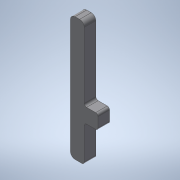
# Autodesk Inventor part: Zlifter
Saved by Autodesk Inventor 2020 (Build 240168000, 168)
## iProperties
Created: 2019-05-25
Part Number: Zlifter
Material: Generic
Document SubType Name: Modeling
Designer: LillaHunden
Density: 1 g/cm^3
Appearance: Default
Author: LillaHunden
Autodesk Inventor part; units mm, degrees
ref_plane "YZ Plane" through (0, 0, 0) normal (1, 0, 0) x (0, 1, 0)
ref_plane "XZ Plane" through (0, 0, 0) normal (0, 1, 0) x (-1, 0, 0)
ref_plane "XY Plane" through (0, 0, 0) normal (0, 0, 1) x (1, 0, 0)
sketch "Sketch1" plane through (0, 0, 0) normal (0, 0, 1) x (1, 0, 0)
  circle A0 centre (-14.5473, 15.1065) radius 1.65 construction
  circle A1 centre (16.4527, 46.1065) radius 1.65 construction
  circle A2 centre (-14.5473, 46.1065) radius 1.65 construction
  circle A3 centre (16.4527, 15.1065) radius 1.65 construction
  circle A4 centre (0.5246, -13.3925) radius 6.1 construction
  circle A5 centre (0.9527, 30.6065) radius 4.765 construction
  circle A6 centre (-32.0049, -58.1419) radius 2.2 construction
  circle A7 centre (-32.0049, -26.1419) radius 2.2 construction
  circle A8 centre (-21.0049, -26.1419) radius 2.2 construction
  circle A9 centre (-32.0049, -42.1419) radius 2.2 construction
  circle A10 centre (-32.0049, 13.8581) radius 2.2 construction
  arc A11 (27.3227, 8.6665) -> (21.7227, 8.6665) centre (24.5227, 8.6665) ccw construction
  line L0 (27.3227, 8.6665) -> (27.3227, 5.6665) construction
  arc A12 (21.7227, 5.6665) -> (27.3227, 5.6665) centre (24.5227, 5.6665) ccw construction
  line L1 (21.7227, 5.6665) -> (21.7227, 8.6665) construction
  arc A13 (-19.8173, 8.6665) -> (-25.4173, 8.6665) centre (-22.6173, 8.6665) ccw construction
  line L2 (-19.8173, 8.6665) -> (-19.8173, 5.6665) construction
  arc A14 (-25.4173, 5.6665) -> (-19.8173, 5.6665) centre (-22.6173, 5.6665) ccw construction
  line L3 (-25.4173, 5.6665) -> (-25.4173, 8.6665) construction
  arc A15 (27.3227, 55.8065) -> (21.7227, 55.8065) centre (24.5227, 55.8065) ccw construction
  line L4 (27.3227, 55.8065) -> (27.3227, 52.8065) construction
  arc A16 (21.7227, 52.8065) -> (27.3227, 52.8065) centre (24.5227, 52.8065) ccw construction
  line L5 (21.7227, 52.8065) -> (21.7227, 55.8065) construction
  arc A17 (-25.4173, 52.8065) -> (-19.8173, 52.8065) centre (-22.6173, 52.8065) ccw construction
  line L6 (-25.4173, 52.8065) -> (-25.4173, 55.8065) construction
  arc A18 (-19.8173, 55.8065) -> (-25.4173, 55.8065) centre (-22.6173, 55.8065) ccw construction
  line L7 (-19.8173, 55.8065) -> (-19.8173, 52.8065) construction
  arc A19 (36.0049, 57.8065) -> (30.0049, 63.8065) centre (30.0049, 57.8065) ccw construction
  line L8 (30.0049, 63.8065) -> (-34.0049, 63.8065) construction
  arc A20 (-34.0049, 63.8065) -> (-40.0049, 57.8065) centre (-34.0049, 57.8065) ccw construction
  line L9 (-40.0049, -59.8065) -> (-40.0049, 57.8065) construction
  arc A21 (-40.0049, -59.8065) -> (-36.0049, -63.8065) centre (-36.0049, -59.8065) ccw construction
  line L10 (-19.1877, -63.8065) -> (-36.0049, -63.8065) construction
  arc A22 (-19.1877, -63.8065) -> (-12.1142, -59.5435) centre (-19.1877, -55.8065) ccw construction
  arc A23 (33.0556, -4.4538) -> (-12.1142, -59.5435) centre (145.8325, -142.9862) ccw construction
  arc A24 (33.0556, -4.4538) -> (36.0049, 1.7503) centre (28.0049, 1.7503) ccw construction
  line L11 (36.0049, 1.7503) -> (36.0049, 57.8065) construction
  line L12 (-36.0049, -63.8065) -> (-30.0709, -63.8065)
  line L13 (-32.0709, 42.9681) -> (-36.0049, 42.9681)
  line L14 (-40.0049, 38.9681) -> (-40.0049, -59.8065)
  line L15 (-26.0709, -19.8799) -> (-18.1973, -19.8799)
  line L16 (-16.1973, -21.8799) -> (-16.1973, -30.4039)
  line L17 (-18.1973, -32.4039) -> (-26.0709, -32.4039)
  line L18 (-40.0049, -31.0336) -> (-40.0049, -21.6758)
  line L19 (-28.0709, -61.8065) -> (-28.0709, -34.4039)
  line L20 (-28.0709, -17.8799) -> (-28.0709, 38.9681)
  arc A25 (-16.1973, -21.8799) -> (-18.1973, -19.8799) centre (-18.1973, -21.8799) ccw
  arc A26 (-18.1973, -32.4039) -> (-16.1973, -30.4039) centre (-18.1973, -30.4039) ccw
  arc A27 (-26.0709, -32.4039) -> (-28.0709, -34.4039) centre (-26.0709, -34.4039) ccw
  arc A28 (-28.0709, -17.8799) -> (-26.0709, -19.8799) centre (-26.0709, -17.8799) ccw
  arc A29 (-40.0049, -59.8065) -> (-36.0049, -63.8065) centre (-36.0049, -59.8065) ccw
  arc A30 (-30.0709, -63.8065) -> (-28.0709, -61.8065) centre (-30.0709, -61.8065) ccw
  arc A31 (-28.0709, 40.9681) -> (-30.0709, 42.9681) centre (-30.0709, 40.9681) ccw
  arc A32 (-36.0049, 42.9681) -> (-40.0049, 38.9681) centre (-36.0049, 38.9681) ccw
  arc A33 (-28.0709, 38.9681) -> (-32.0709, 42.9681) centre (-32.0709, 38.9681) ccw
  point P0 (0, 0)
  point P1 (-16.1973, -26.1419)
  point P2 (-34.0379, -63.8065)
  dimension "d0" = 2
  dimension "d1" = 2
  dimension "d2" = 4
  constraints: 20 point on circle, 18 end point, 17 tangent, 9 centre point, 6 equal radius, 5 parallel, 5 point on line, 3 perpendicular, 2 horizontal, 1 horizontal alignment, 1 midpoint
  measures "d0" radius of A25
  measures "d1" radius of A30
  measures "d2" radius of A32
extrude "Extrusion1" add sketch "Sketch1" along normal blind 10
sketch "Sketch2" plane through (-40.0049, -59.8065, 0) normal (-1, 0, 0) x (0, 0, 1)
  line L0 (0, 98.7746) -> (0, 0) projected
  line L1 (0, 0) -> (10, 0) projected
  line L2 (10, 98.7746) -> (10, 0) projected
  line L3 (0, 98.7746) -> (10, 98.7746) projected
  point P0 (0, 59.8065)
extrude "Extrusion2" add sketch "Sketch2" along normal blind 49.75
sketch "Sketch3" plane through (0, 0, 10) normal (0, 0, 1) x (1, 0, 0)
  circle A0 centre (-21.0049, -26.1419) radius 2.2 projected
  circle A1 centre (-32.0049, 13.8581) radius 2.2 projected
  circle A2 centre (-32.0049, -26.1419) radius 2.2 projected
  circle A3 centre (-32.0049, -58.1419) radius 2.2 projected
  circle A4 centre (-32.0049, -42.1419) radius 2.2 projected
  point P0 (0, 0)
extrude "Extrusion3" cut sketch "Sketch3" against normal through all
sketch "Sketch4" plane through (-89.7549, -59.8065, 0) normal (-1, 0, 0) x (0, 0, 1)
  line L0 (5.5, 98.7746) -> (0, 98.7746)
  line L1 (0, 98.7746) -> (0, 0)
  line L2 (0, 0) -> (5.5, 0)
  line L3 (5.5, 0) -> (5.5, 98.7746)
  line L4 (10, 0) -> (10, 98.7746) projected
  point P0 (0, 59.8065)
  dimension "d9" = 4.5
  constraints: 8 end point, 2 parallel, 1 horizontal, 1 perpendicular
  measures "d9" distance between parallel lines of L3 L4
extrude "Extrusion4" cut sketch "Sketch4" against normal blind 27
sketch "Sketch5" plane through (0, 0, 10) normal (0, 0, 1) x (1, 0, 0)
  circle A0 centre (-32.0049, 38.3346) radius 2.2
  circle A1 centre (-32.0049, 13.8581) radius 2.2 projected
  point P0 (0, 0)
  dimension "d12" = 4.4
  constraints: 1 centre point, 1 vertical alignment
  measures "d12" diameter of A0
extrude "Extrusion5" cut sketch "Sketch5" against normal through all contours A0
body "Solid1"
